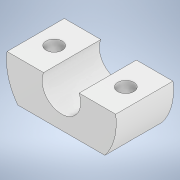
# Autodesk Inventor part: SU22_3DP_EU_Sub_sn
Saved by Autodesk Inventor 2022 (Build 260153000, 153)
## iProperties
Created: 2022-06-28
Part Number: SU22_3DP_EU_Sub_sn
Material: ABS プラスチック
Document SubType Name: Modeling
Designer: 中島 青蔵
Density: 1.06 g/cm^3
Appearance: 滑らか - 白
Author: 中島 青蔵
Autodesk Inventor part; units mm, degrees
ref_plane "YZ Plane" through (0, 0, 0) normal (1, 0, 0) x (0, 1, 0)
ref_plane "XZ Plane" through (0, 0, 0) normal (0, 1, 0) x (-1, 0, 0)
ref_plane "XY Plane" through (0, 0, 0) normal (0, 0, 1) x (1, 0, 0)
sketch "スケッチ1" plane through (0, 0, 0) normal (0, 0, 1) x (1, 0, 0)
  circle A0 centre (0, 0) radius 4.05
  circle A1 centre (0, 0) radius 11.5
  line L0 (-1.2, 1.6) -> (1.2, 1.6)
  line L1 (11.3882, 1.6) -> (1.2, 1.6)
  line L2 (-1.2, 1.6) -> (-11.3882, 1.6)
  circle A2 centre (0, 0) radius 2
  line L3 (9.1241, -7) -> (-9.1241, -7)
  point P0 (3.7206, 1.6)
  point P1 (-3.7206, 1.6)
  dimension "d0" = 8.1
  dimension "d1" = 23
  dimension "d3" = 4
  dimension "d4" = 2.4
  dimension "d5" = 7
  constraints: 8 end point, 6 point on circle, 3 centre point, 3 coincident, 2 point on line, 1 horizontal, 1 parallel
  measures "d0" diameter of A0
  measures "d1" diameter of A1
  measures "d3" diameter of A2
  measures "d4" distance of L0.start L0.end
  measures "d5" distance from line of L3 point (0, 0)
extrude "押し出し1" add sketch "スケッチ1" along normal blind 12 contours A0 L1 A1 L3 L2
sketch "スケッチ3" plane through (-11.3882, 1.6, 0) normal (0, 1, 0) x (1, 0, 0)
  line L0 (22.7763, 0) -> (15.1087, 0) projected
  line L1 (7.6676, 0) -> (0, 0) projected
  point P0 (11.3882, 0)
  point P1 (3.8882, -6)
  point P2 (18.8882, -6)
  dimension "d8" = 6
  dimension "d9" = 7.5
  dimension "d10" = 7.5
  dimension "d11" = 6
  measures "d8" distance from line of L0 point (18.888, -6)
  measures "d9" horizontal distance of point (11.388, 0) point (18.888, -6)
  measures "d10" horizontal distance of point (11.388, 0) point (3.888, -6)
  measures "d11" distance from line of L1 point (3.888, -6)
hole "穴1" at (-7.5, 1.6, 6) at (7.5, 1.6, 6) direction (0, -1, 0) diameter 3.4 end through all
equation "\"d10\" = d9"
equation "\"d11\" = d8"
